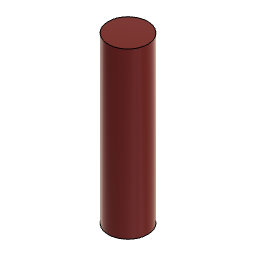
tvcf3z (Autodesk Fusion 360 archive; units mm, degrees)
design "Motor24mm"
Autodesk Fusion 360 part; units mm, degrees
sketch "Sketch1" plane through (0, 0, 0) normal (0, 0, 1) x (1, 0, 0)
  circle A0 centre (0, 0) radius 12
  dimension "d1" = 24
  constraint coincident A0.centre origin
  measures "d1" diameter of A0
extrude "Extrude1" add sketch "Sketch1" along normal blind 100

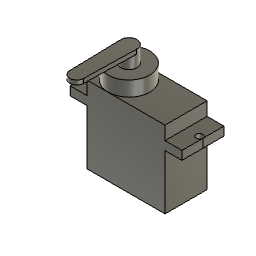
design "MicroServo"
Autodesk Fusion 360 part; units mm, degrees
sketch "Sketch1" plane through (0, 0, 0) normal (0, 0, 1) x (1, 0, 0)
  line L0 (-11.3, 6.1) -> (11.3, 6.1)
  line L1 (11.3, 6.1) -> (11.3, -6.1)
  line L2 (11.3, -6.1) -> (-11.3, -6.1)
  line L3 (-11.3, -6.1) -> (-11.3, 6.1)
  line L4 (-11.3, 6.1) -> (11.3, -6.1) construction
  line L5 (11.3, 6.1) -> (-11.3, -6.1) construction
  dimension "d3" = 22.6
  dimension "d4" = 12.2
  constraint horizontal L0
  constraint perpendicular L0 L1
  constraint parallel L0 L2
  constraint parallel L1 L3
  constraint coincident L4 origin
  constraint coincident L5 origin
  measures "d3" distance of L1.end L2.end
  measures "d4" distance of L0.end L1.end
extrude "Extrude1" add sketch "Sketch1" along normal blind 15.9 makes body 1
sketch "Sketch2" plane through (0, 0, 15.9) normal (0, 0, 1) x (-1, 0, 0)
  line L0 (11.3, 6.1) -> (-11.3, 6.1)
  line L1 (-11.3, 6.1) -> (-11.3, -6.1)
  line L2 (-11.3, -6.1) -> (11.3, -6.1)
  line L3 (11.3, -6.1) -> (11.3, 6.1)
  line L4 (-11.3, -6.1) -> (-16.21, -6.1)
  line L5 (-16.21, -6.1) -> (-16.21, 6.1)
  line L6 (-16.21, 6.1) -> (-11.3, 6.1)
  line L7 (-11.3, 6.1) -> (-11.3, -6.1)
  circle A0 centre (-15.21, 0) radius 1
  line L8 (0, -6.1) -> (0, 6.1) construction
  line L9 (11.3, -6.1) -> (16.21, -6.1)
  line L10 (16.21, -6.1) -> (16.21, 6.1)
  line L11 (16.21, 6.1) -> (11.3, 6.1)
  circle A1 centre (15.21, 0) radius 1
  dimension "d7" = 4.91
  dimension "d8" = 2
  constraint horizontal L4
  constraint vertical L5
  constraint horizontal L6
  constraint vertical L7
  constraint coincident L1.end L2.start
  constraint midpoint L2 L8.start
  constraint midpoint L0 L8.end
  constraint symmetric L1.end L8 L2.end
  constraint symmetric L4.end L8 L9.end
  constraint symmetric L5.end L8 L10.end
  constraint symmetric L0.end L8 L0.start
  constraint symmetric A0 L8 A1
  measures "d7" distance of L1.end L4.end
  measures "d8" diameter of A0
extrude "Extrude2" add sketch "Sketch2" along normal blind 2.5 separate body contours L3 L9 L10 L11 | L1 L4 L5 L6 L7 makes body 2 at (14.1182, 4.377, 15.9) makes body 3 at (-14.1182, 4.377, 15.9)
extrude "Extrude3" add 1 faces at (-3.7667, 2.0333, 15.9) along direction (0, 0, 1) blind 6.4 on bodies 1 bodies 1 2 3
sketch "Sketch3" plane through (0, 0, 22.3) normal (0, 0, 1) x (-1, 0, 0)
  line L0 (11.3, 6.1) -> (-11.3, 6.1)
  line L1 (-11.3, 6.1) -> (-11.3, -6.1)
  line L2 (-11.3, -6.1) -> (11.3, -6.1)
  line L3 (11.3, -6.1) -> (11.3, 6.1)
  circle A0 centre (5.24, 0.04) radius 6.06
  circle A1 centre (5.24, 0.04) radius 2.35
  dimension "d13" = 6.06
  dimension "d14" = 4.7
  constraint tangent L3 A0
  constraint tangent L0 A0
  constraint concentric A0 A1
  measures "d13" radius of A0
  measures "d14" diameter of A1
extrude "Extrude4" add sketch "Sketch3" along normal blind 4.3 separate body contours A0 makes body 4
extrude "Extrude5" add sketch "Sketch3" along normal blind 9 contours A1 bodies 4 1
sketch "Sketch4" plane through (0, 0, 31.3) normal (0, 0, 1) x (-1, 0, 0)
  circle A0 centre (5.24, 0.04) radius 2.35
  line L0 (5.24, 0.04) -> (5.24, -2.31) construction
  line L1 (5.24, -2.31) -> (5.24, 17.19) construction
  circle A1 centre (5.24, 15.19) radius 2
  line L2 (5.24, 0.04) -> (7.59, 0.04) construction
  line L3 (5.24, 0.04) -> (2.89, 0.04) construction
  line L4 (5.24, 15.19) -> (7.24, 15.19) construction
  line L5 (5.24, 15.19) -> (3.24, 15.19) construction
  line L6 (7.59, 0.04) -> (7.24, 15.19)
  line L7 (2.89, 0.04) -> (3.24, 15.19)
  dimension "d19" = 19.5
  dimension "d20" = 4
  constraint coincident A0.centre L0.start
  constraint coincident A0 L0.end
  constraint vertical L0
  constraint parallel L0 L1
  constraint coincident L1.end A1
  constraint coincident A0 L2.end
  constraint perpendicular L1 L2
  constraint coincident A0 L3.end
  constraint perpendicular L0 L3
  constraint coincident A1.centre L4.start
  constraint coincident A1 L4.end
  constraint perpendicular L1 L4
  constraint coincident A1 L5.end
  constraint perpendicular L1 L5
  measures "d19" distance of L0.end L1.end
  measures "d20" diameter of A1
extrude "Extrude6" add sketch "Sketch4" against normal blind 1.25 separate body contours A0 A1 L6 L7 | A1 makes body 5
split "Split1" by plane through (0, 0, 26.6) normal (0, 0, 1) bodies 4 makes body 6 at (-7.5783, 0.194, 28.1667)
combine "Combine1" operation add target body 6 tool bodies 5 result as body 7 in component "ServoArm"
delete_body "RemoveBody2" bodies 6
copy_body "Body->Comp1" bodies 4 removing the originals makes body 8 in component "ServoBody"
component "ServoArm" placed x (1, 0, 0) y (0, 1, 0) z (0, 0, 1) at (0, 0, 0)
component "ServoBody" placed x (1, 0, 0) y (0, 1, 0) z (0, 0, 1) at (0, 0, 0)
equation "base_height = 12.2 mm"
equation "base_width = 22.6 mm"
equation "d3 = base_width"
equation "d4 = base_height"
equation "d5 = 18.4 mm - 2.5 mm"
equation "d7 = ( ( 32.15 - 22.33 ) / 2 ) * 1 mm"
equation "d11 = 22.3 mm - 15.9 mm"
equation "d15 = 26.61 mm - 22.31 mm"
equation "d17 = 31.51 mm - 22.51 mm"
